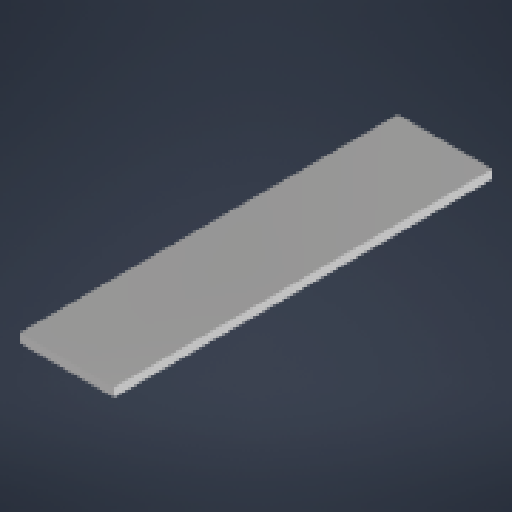
# Autodesk Inventor part: dot matrix cover
Saved by Autodesk Inventor 2024 (Build 280153000, 153)
## iProperties
Created: 2023-07-17
Part Number: dot matrix cover
Material: 유리, 젖빛
Document SubType Name: Modeling
Designer: wodyd
Mass: 26.7878 g
Surface Area: 91.52 cm^2
Volume: 12.288 cm^3
Density: 2.18 g/cm^3
Appearance: 젖빛 - 흰색
Author: wodyd
Autodesk Inventor part; units mm, degrees
ref_plane "YZ Plane" through (0, 0, 0) normal (1, 0, 0) x (0, 1, 0)
ref_plane "XZ Plane" through (0, 0, 0) normal (0, 1, 0) x (-1, 0, 0)
ref_plane "XY Plane" through (0, 0, 0) normal (0, 0, 1) x (1, 0, 0)
sketch "스케치1" plane through (0, 0, 0) normal (0, 0, 1) x (1, 0, 0)
  line L0 (0, 0) -> (32, 0)
  line L1 (32, 0) -> (32, -3)
  line L2 (32, -3) -> (0, -3)
  line L3 (0, -3) -> (0, 0)
  dimension "d0" = 32
  dimension "d1" = 3
  constraints: 8 end point, 2 parallel, 1 horizontal, 1 perpendicular
  measures "d0" distance of L1.end L2.end
  measures "d1" distance of L0.end L1.end
extrude "돌출1" add sketch "스케치1" along normal blind 128
